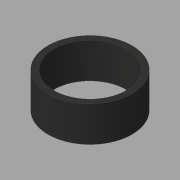
# Autodesk Inventor part: Tube grip
Saved by Autodesk Inventor 2017 (Build 210142000, 142)
## iProperties
Created: 2017-01-17
Part Number: Tube grip
Material: Rubber, Silicone
Document SubType Name: Modeling
Designer: qupec
Density: 1.25 g/cm^3
Appearance: Rubber - Black
Mass: 1.25562 g
Surface Area: 14.7642 cm^2
Volume: 1.00449 cm^3
Author: qupec
Autodesk Inventor part; units mm, degrees
ref_plane "YZ Plane" through (0, 0, 0) normal (1, 0, 0) x (0, 1, 0)
ref_plane "XZ Plane" through (0, 0, 0) normal (0, 1, 0) x (-1, 0, 0)
ref_plane "XY Plane" through (0, 0, 0) normal (0, 0, 1) x (1, 0, 0)
sketch "Sketch1" plane through (0, 0, 0) normal (0, 1, 0) x (-1, 0, 0)
  circle A0 centre (0, 0) radius 11.3665
  circle A1 centre (0, 0) radius 9.779
  dimension "d0" = 22.733
  dimension "d1" = 19.558
  dimension "d4" = 1.5875
  constraints: 2 centre point, 2 coincident
  measures "d0" diameter of A0
  measures "d1" diameter of A1
  measures "d4" radial gap between concentric circles of A0 A1
extrude "Extrusion1" add sketch "Sketch1" along normal blind 9.525
body "Solid1"
